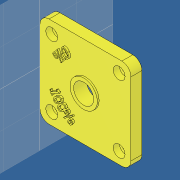
# Autodesk Inventor part: Schalter_Platte_0-100
Saved by Autodesk Inventor 2019 (Build 230136000, 136)
## iProperties
Created: 2020-08-07
Part Number: Schalter_Platte_0-100
Material: Generisch
Document SubType Name: Modeling
Designer: Stefan
Mass: 13.8842 g
Surface Area: 66.8299 cm^2
Volume: 13.8842 cm^3
Density: 1 g/cm^3
Appearance: Glatt - Gelb
Author: Stefan
Autodesk Inventor part; units mm, degrees
ref_plane "YZ Plane" through (0, 0, 0) normal (1, 0, 0) x (0, 1, 0)
ref_plane "XZ Plane" through (0, 0, 0) normal (0, 1, 0) x (-1, 0, 0)
ref_plane "XY Plane" through (0, 0, 0) normal (0, 0, 1) x (1, 0, 0)
sketch "Skizze1" plane through (0, 0, 0) normal (0, 0, 1) x (1, 0, 0)
  line L0 (-20, 25) -> (20, 25)
  line L1 (25, 20) -> (25, -20)
  line L2 (20, -25) -> (-20, -25)
  line L3 (-25, -20) -> (-25, 20)
  line L4 (-25, 25) -> (25, -25) construction
  line L5 (25, 25) -> (-25, -25) construction
  arc A0 (25, 20) -> (20, 25) centre (20, 20) ccw
  arc A1 (20, -25) -> (25, -20) centre (20, -20) ccw
  arc A2 (-25, -20) -> (-20, -25) centre (-20, -20) ccw
  arc A3 (-20, 25) -> (-25, 20) centre (-20, 20) ccw
  circle A4 centre (0, 0) radius 5.5
  circle A5 centre (0, 0) radius 15 construction
  circle A6 centre (0, 0) radius 7.5
  spline S0 degree 2 poles (-11.4587, 13.3233) (-12.2394, 14.4188) (-12.3337, 15.8989) (-11.6705, 16.3715) knots 0 0 0 1 2 2 2
  spline S1 degree 2 poles (-11.6705, 16.3715) (-10.9973, 16.8511) (-9.6217, 16.2542) (-8.8575, 15.1817) knots 0 0 0 1 2 2 2
  spline S2 degree 2 poles (-8.8575, 15.1817) (-8.0722, 14.0796) (-7.9825, 12.6061) (-8.6491, 12.1312) knots 0 0 0 1 2 2 2
  spline S3 degree 2 poles (-8.6491, 12.1312) (-9.3189, 11.6539) (-10.7016, 12.2607) (-11.4587, 13.3233) knots 0 0 0 1 2 2 2
  spline S4 degree 2 poles (-11.6433, 15.0625) (-11.579, 14.8048) (-11.203, 14.1374) (-10.9044, 13.7183) knots 0 0 0 1 2 2 2
  spline S5 degree 2 poles (-10.9044, 13.7183) (-10.6057, 13.2992) (-10.1, 12.7291) (-9.8694, 12.58) knots 0 0 0 1 2 2 2
  spline S6 degree 2 poles (-9.8694, 12.58) (-9.6388, 12.4309) (-9.1989, 12.421) (-8.9712, 12.5832) knots 0 0 0 1 2 2 2
  spline S7 degree 2 poles (-8.9712, 12.5832) (-8.7435, 12.7455) (-8.6026, 13.1692) (-8.6697, 13.4449) knots 0 0 0 1 2 2 2
  spline S8 degree 2 poles (-8.6697, 13.4449) (-8.7353, 13.7115) (-9.1274, 14.3874) (-9.4119, 14.7867) knots 0 0 0 1 2 2 2
  spline S9 degree 2 poles (-9.4119, 14.7867) (-9.7175, 15.2157) (-10.1795, 15.7522) (-10.4252, 15.9155) knots 0 0 0 1 2 2 2
  spline S10 degree 2 poles (-10.4252, 15.9155) (-10.6548, 16.0703) (-11.1108, 16.0887) (-11.3484, 15.9194) knots 0 0 0 1 2 2 2
  spline S11 degree 2 poles (-11.3484, 15.9194) (-11.5727, 15.7595) (-11.7136, 15.3357) (-11.6433, 15.0625) knots 0 0 0 1 2 2 2
  spline S12 degree 2 poles (-16.2559, 9.5557) (-16.8363, 10.0365) (-17.0102, 10.9698) (-16.6431, 11.4129) knots 0 0 0 1 2 2 2
  spline S13 degree 2 poles (-16.6431, 11.4129) (-16.2708, 11.8622) (-15.3204, 11.8535) (-14.7463, 11.3778) knots 0 0 0 1 2 2 2
  spline S14 degree 2 poles (-14.7463, 11.3778) (-14.1691, 10.8996) (-13.9946, 9.9606) (-14.3591, 9.5207) knots 0 0 0 1 2 2 2
  spline S15 degree 2 poles (-14.3591, 9.5207) (-14.734, 9.0682) (-15.6818, 9.08) (-16.2559, 9.5557) knots 0 0 0 1 2 2 2
  spline S16 degree 2 poles (-12.2087, 10.954) (-12.7891, 11.4348) (-12.9629, 12.3681) (-12.5959, 12.8112) knots 0 0 0 1 2 2 2
  spline S17 degree 2 poles (-12.5959, 12.8112) (-12.2236, 13.2605) (-11.2732, 13.2518) (-10.6991, 12.7762) knots 0 0 0 1 2 2 2
  spline S18 degree 2 poles (-10.6991, 12.7762) (-10.1218, 12.298) (-9.9474, 11.3589) (-10.3119, 10.919) knots 0 0 0 1 2 2 2
  spline S19 degree 2 poles (-10.3119, 10.919) (-10.6867, 10.4666) (-11.6346, 10.4784) (-12.2087, 10.954) knots 0 0 0 1 2 2 2
  line L6 (-12.5654, 8.345) -> (-14.7458, 13.5505)
  line L7 (-14.7458, 13.5505) -> (-14.3916, 13.978)
  line L8 (-14.3916, 13.978) -> (-12.2113, 8.7725)
  line L9 (-12.2113, 8.7725) -> (-12.5654, 8.345)
  spline S20 degree 2 poles (-11.8287, 11.4127) (-11.4325, 11.0844) (-10.8774, 10.935) (-10.6577, 11.2002) knots 0 0 0 1 2 2 2
  spline S21 degree 2 poles (-10.6577, 11.2002) (-10.438, 11.4654) (-10.6916, 11.9913) (-11.0816, 12.3144) knots 0 0 0 1 2 2 2
  spline S22 degree 2 poles (-11.0816, 12.3144) (-11.4717, 12.6375) (-12.0252, 12.8014) (-12.2552, 12.5237) knots 0 0 0 1 2 2 2
  spline S23 degree 2 poles (-12.2552, 12.5237) (-12.475, 12.2585) (-12.2187, 11.7358) (-11.8287, 11.4127) knots 0 0 0 1 2 2 2
  spline S24 degree 2 poles (-15.8759, 10.0143) (-15.4797, 9.686) (-14.9247, 9.5367) (-14.7049, 9.8019) knots 0 0 0 1 2 2 2
  spline S25 degree 2 poles (-14.7049, 9.8019) (-14.4852, 10.0671) (-14.7388, 10.5929) (-15.1289, 10.9161) knots 0 0 0 1 2 2 2
  spline S26 degree 2 poles (-15.1289, 10.9161) (-15.5189, 11.2392) (-16.0724, 11.4031) (-16.3025, 11.1254) knots 0 0 0 1 2 2 2
  spline S27 degree 2 poles (-16.3025, 11.1254) (-16.5222, 10.8602) (-16.266, 10.3375) (-15.8759, 10.0143) knots 0 0 0 1 2 2 2
  line L10 (-17.6091, -9.5741) -> (-18.6305, -7.359)
  line L11 (-18.6305, -7.359) -> (-18.1669, -7.1453)
  line L12 (-18.1669, -7.1453) -> (-17.7868, -7.9695)
  line L13 (-17.7868, -7.9695) -> (-14.7438, -6.5664)
  line L14 (-14.7438, -6.5664) -> (-15.1239, -5.7421)
  line L15 (-15.1239, -5.7421) -> (-14.7081, -5.5504)
  spline S28 degree 2 poles (-14.7081, -5.5504) (-14.4926, -6.0177) (-14.0241, -6.3371) (-13.6426, -6.1969) knots 0 0 0 1 2 2 2
  line L16 (-13.6426, -6.1969) -> (-13.4254, -6.6679)
  line L17 (-13.4254, -6.6679) -> (-17.5171, -8.5545)
  line L18 (-17.5171, -8.5545) -> (-17.1455, -9.3603)
  line L19 (-17.1455, -9.3603) -> (-17.6091, -9.5741)
  spline S29 degree 2 poles (-13.3233, -11.4587) (-14.4188, -12.2394) (-15.8989, -12.3337) (-16.3715, -11.6705) knots 0 0 0 1 2 2 2
  spline S30 degree 2 poles (-16.3715, -11.6705) (-16.8511, -10.9973) (-16.2542, -9.6217) (-15.1817, -8.8575) knots 0 0 0 1 2 2 2
  spline S31 degree 2 poles (-15.1817, -8.8575) (-14.0796, -8.0722) (-12.6061, -7.9825) (-12.1312, -8.6491) knots 0 0 0 1 2 2 2
  spline S32 degree 2 poles (-12.1312, -8.6491) (-11.6539, -9.3189) (-12.2607, -10.7016) (-13.3233, -11.4587) knots 0 0 0 1 2 2 2
  spline S33 degree 2 poles (-15.0625, -11.6433) (-14.8048, -11.579) (-14.1374, -11.203) (-13.7183, -10.9044) knots 0 0 0 1 2 2 2
  spline S34 degree 2 poles (-13.7183, -10.9044) (-13.2992, -10.6057) (-12.7291, -10.1) (-12.58, -9.8694) knots 0 0 0 1 2 2 2
  spline S35 degree 2 poles (-12.58, -9.8694) (-12.4309, -9.6388) (-12.421, -9.1989) (-12.5832, -8.9712) knots 0 0 0 1 2 2 2
  spline S36 degree 2 poles (-12.5832, -8.9712) (-12.7455, -8.7435) (-13.1692, -8.6026) (-13.4449, -8.6697) knots 0 0 0 1 2 2 2
  spline S37 degree 2 poles (-13.4449, -8.6697) (-13.7115, -8.7353) (-14.3874, -9.1274) (-14.7867, -9.4119) knots 0 0 0 1 2 2 2
  spline S38 degree 2 poles (-14.7867, -9.4119) (-15.2157, -9.7175) (-15.7522, -10.1795) (-15.9155, -10.4252) knots 0 0 0 1 2 2 2
  spline S39 degree 2 poles (-15.9155, -10.4252) (-16.0703, -10.6548) (-16.0887, -11.1108) (-15.9194, -11.3484) knots 0 0 0 1 2 2 2
  spline S40 degree 2 poles (-15.9194, -11.3484) (-15.7595, -11.5727) (-15.3357, -11.7136) (-15.0625, -11.6433) knots 0 0 0 1 2 2 2
  spline S41 degree 2 poles (-10.9599, -13.7365) (-11.8912, -14.7073) (-13.3279, -15.0752) (-13.9156, -14.5114) knots 0 0 0 1 2 2 2
  spline S42 degree 2 poles (-13.9156, -14.5114) (-14.5121, -13.9392) (-14.1814, -12.4766) (-13.2697, -11.5263) knots 0 0 0 1 2 2 2
  spline S43 degree 2 poles (-13.2697, -11.5263) (-12.3328, -10.5497) (-10.9018, -10.1875) (-10.3111, -10.7542) knots 0 0 0 1 2 2 2
  spline S44 degree 2 poles (-10.3111, -10.7542) (-9.7176, -11.3236) (-10.0567, -12.795) (-10.9599, -13.7365) knots 0 0 0 1 2 2 2
  spline S45 degree 2 poles (-12.6345, -14.2412) (-12.3932, -14.1302) (-11.8074, -13.6366) (-11.4511, -13.2653) knots 0 0 0 1 2 2 2
  spline S46 degree 2 poles (-11.4511, -13.2653) (-11.0949, -12.8939) (-10.6289, -12.291) (-10.5252, -12.0367) knots 0 0 0 1 2 2 2
  spline S47 degree 2 poles (-10.5252, -12.0367) (-10.4216, -11.7824) (-10.4937, -11.3483) (-10.6954, -11.1547) knots 0 0 0 1 2 2 2
  spline S48 degree 2 poles (-10.6954, -11.1547) (-10.8972, -10.9612) (-11.3397, -10.9016) (-11.5981, -11.0187) knots 0 0 0 1 2 2 2
  spline S49 degree 2 poles (-11.5981, -11.0187) (-11.8479, -11.1328) (-12.4391, -11.6437) (-12.7785, -11.9975) knots 0 0 0 1 2 2 2
  spline S50 degree 2 poles (-12.7785, -11.9975) (-13.1432, -12.3776) (-13.5844, -12.9313) (-13.6992, -13.203) knots 0 0 0 1 2 2 2
  spline S51 degree 2 poles (-13.6992, -13.203) (-13.8085, -13.4575) (-13.7418, -13.9089) (-13.5313, -14.1108) knots 0 0 0 1 2 2 2
  spline S52 degree 2 poles (-13.5313, -14.1108) (-13.3325, -14.3016) (-12.8899, -14.3612) (-12.6345, -14.2412) knots 0 0 0 1 2 2 2
  spline S53 degree 2 poles (-6.366, -17.7494) (-6.7305, -18.409) (-7.6152, -18.7534) (-8.1188, -18.4752) knots 0 0 0 1 2 2 2
  spline S54 degree 2 poles (-8.1188, -18.4752) (-8.6294, -18.193) (-8.7977, -17.2575) (-8.4371, -16.6049) knots 0 0 0 1 2 2 2
  spline S55 degree 2 poles (-8.4371, -16.6049) (-8.0745, -15.9488) (-7.1843, -15.6029) (-6.6843, -15.8792) knots 0 0 0 1 2 2 2
  spline S56 degree 2 poles (-6.6843, -15.8792) (-6.17, -16.1633) (-6.0054, -17.0968) (-6.366, -17.7494) knots 0 0 0 1 2 2 2
  spline S57 degree 2 poles (-8.4925, -14.0328) (-8.857, -14.6924) (-9.7417, -15.0369) (-10.2453, -14.7586) knots 0 0 0 1 2 2 2
  spline S58 degree 2 poles (-10.2453, -14.7586) (-10.756, -14.4764) (-10.9242, -13.5409) (-10.5637, -12.8884) knots 0 0 0 1 2 2 2
  spline S59 degree 2 poles (-10.5637, -12.8884) (-10.2011, -12.2323) (-9.3109, -11.8863) (-8.8109, -12.1626) knots 0 0 0 1 2 2 2
  spline S60 degree 2 poles (-8.8109, -12.1626) (-8.2966, -12.4467) (-8.132, -13.3803) (-8.4925, -14.0328) knots 0 0 0 1 2 2 2
  line L20 (-5.8627, -13.8981) -> (-10.572, -17.0085)
  line L21 (-10.572, -17.0085) -> (-11.0578, -16.74)
  line L22 (-11.0578, -16.74) -> (-6.3486, -13.6296)
  line L23 (-6.3486, -13.6296) -> (-5.8627, -13.8981)
  spline S61 degree 2 poles (-9.0139, -13.7447) (-8.765, -13.2943) (-8.7214, -12.7212) (-9.0229, -12.5547) knots 0 0 0 1 2 2 2
  spline S62 degree 2 poles (-9.0229, -12.5547) (-9.3243, -12.3881) (-9.7938, -12.7351) (-10.0388, -13.1784) knots 0 0 0 1 2 2 2
  spline S63 degree 2 poles (-10.0388, -13.1784) (-10.2837, -13.6217) (-10.3419, -14.196) (-10.0262, -14.3704) knots 0 0 0 1 2 2 2
  spline S64 degree 2 poles (-10.0262, -14.3704) (-9.7248, -14.537) (-9.2588, -14.188) (-9.0139, -13.7447) knots 0 0 0 1 2 2 2
  spline S65 degree 2 poles (-6.8873, -17.4613) (-6.6384, -17.0109) (-6.5948, -16.4378) (-6.8963, -16.2712) knots 0 0 0 1 2 2 2
  spline S66 degree 2 poles (-6.8963, -16.2712) (-7.1977, -16.1047) (-7.6672, -16.4517) (-7.9122, -16.895) knots 0 0 0 1 2 2 2
  spline S67 degree 2 poles (-7.9122, -16.895) (-8.1572, -17.3383) (-8.2153, -17.9126) (-7.8997, -18.087) knots 0 0 0 1 2 2 2
  spline S68 degree 2 poles (-7.8997, -18.087) (-7.5982, -18.2536) (-7.1322, -17.9046) (-6.8873, -17.4613) knots 0 0 0 1 2 2 2
  point P0 (18.5, 18.5)
  point P1 (18.5, -18.5)
  point P2 (-18.5, -18.5)
  point P3 (-18.5, 18.5)
  dimension "d0" = 50
  dimension "d1" = 50
  dimension "d2" = 5
  dimension "d3" = 37
  dimension "d4" = 11
  dimension "d5" = 30
  dimension "d6" = 15
  constraints: 12 end point, 12 point on line, 8 point on circle, 8 tangent, 7 centre point, 4 coincident, 4 midpoint, 3 equal radius, 2 horizontal alignment, 2 parallel, 1 horizontal, 1 perpendicular, 1 vertical alignment, 2 other
  measures "d0" distance of L5.start L4.end
  measures "d1" distance of L4.start L5.start
  measures "d2" radius of A0
  measures "d3" distance of point (18.5, -18.5) point (18.5, 18.5)
  measures "d4" diameter of A4
  measures "d5" diameter of A5
  measures "d6" diameter of A6
extrude "Extrusion1" add sketch "Skizze1" against normal blind 6 contours L0 A0 L1 A1 L2 A2 L3 A3 | A6 | S0 S1 S2 S3 S18 S17 | S17 S18 S3 | S3 S18 S19 S16 S17 | S11 S10 S9 S8 S7 S6 S5 S4 | S12 S13 S14 S15 | L6 L7 L8 L9 | S23 S22 S21 S20 | S27 S26 S25 S24 | L10 L11 L12 L13 L14 L15 S28 L16 L17 L18 L19 | S29 S30 S31 S32 | S40 S39 S38 S37 S36 S35 S34 S33 | S41 S42 S43 S44 S59 S58 | S58 S59 S44 | S44 S59 S60 S57 S58 | S52 S51 S50 S49 S48 S47 S46 S45 | S53 S54 S55 S56 | L20 L21 L22 L23 | S64 S63 S62 S61 | S68 S67 S66 S65
extrude "Extrusion2" add sketch "Skizze1" along normal blind 1 contours A6
emboss "Prägen1" sketch "Skizze1" operation add depth 1 direction (0, 0, -1) contours S0 S1 S2 S3 S18 S17 | S17 S18 S3 | S3 S18 S19 S16 S17 | S12 S13 S14 S15 | L6 L7 L8 L9 | L10 L11 L12 L13 L14 L15 S28 L16 L17 L18 L19 | S29 S30 S31 S32 | S41 S42 S43 S44 S59 S58 | S58 S59 S44 | S44 S59 S60 S57 S58 | S53 S54 S55 S56 | L20 L21 L22 L23
hole "Bohrung1" at (18.5, -18.5, 0) at (-18.5, 18.5, 0) at (18.5, 18.5, 0) at (-18.5, -18.5, 0) direction (0, 0, -1) diameter 3.4 end through all counterbore diameter 6.5 counterbore depth 3.4 clearance for "Inbusschraube DIN EN ISO 4762" size "M3" standard "DIN"
equation "\"d1\" = d0"
